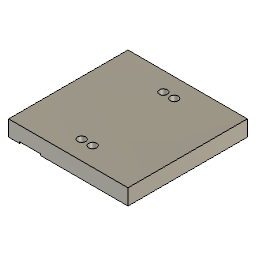
sample_stage (Autodesk Fusion 360 design; units mm, degrees)
part number: 2025-09-14-20-17-25-406
Autodesk Fusion 360 part; units mm, degrees
sketch "Sketch1" plane through (0, 0, 0) normal (0, 1, 0) x (1, 0, 0)
  line L0 (-30, -4) -> (30, -4)
  line L1 (30, -4) -> (30, 4)
  line L2 (30, 4) -> (-30, 4)
  line L3 (-30, 4) -> (-30, -4)
  line L4 (-30, -4) -> (30, 4) construction
  line L5 (30, -4) -> (-30, 4) construction
  line L6 (-30, 4) -> (-20, 4)
  line L7 (-20, 4) -> (-20, 14.75)
  line L8 (-20, 14.75) -> (-30, 14.75)
  line L9 (-30, 14.75) -> (-30, 4)
  line L10 (30, 4) -> (20, 4)
  line L11 (20, 4) -> (20, 14.75)
  line L12 (20, 14.75) -> (30, 14.75)
  line L13 (30, 14.75) -> (30, 4)
  dimension "d1" = 8
  dimension "d2" = 18.75
  dimension "d4" = 10
  dimension "d23" = 60
  constraint horizontal L0
  constraint perpendicular L0 L1
  constraint parallel L0 L2
  constraint parallel L1 L3
  constraint coincident L4 origin
  constraint coincident L5 origin
  constraint horizontal L6
  constraint vertical L7
  constraint horizontal L8
  constraint vertical L9
  constraint horizontal L10
  constraint vertical L11
  constraint horizontal L12
  constraint vertical L13
  constraint equal L8 L12
  constraint equal L9 L11
  measures "d1" distance of L0.end L1.end
  measures "d2" distance of L0 L12
  measures "d4" distance of L11.end L12.end
  measures "d23" distance of L0.start L0.end
extrude "Extrude1" add sketch "Sketch1" along normal mid plane 60 contours L0 L1 L2 L3 L6 L10
sketch "Sketch2" plane through (0, 0, 4) normal (0, 0, 1) x (-1, 0, 0)
  line L0 (-30, 30) -> (-30, -30)
  line L1 (-30, -30) -> (30, -30)
  line L2 (30, -30) -> (30, 30)
  line L3 (30, 30) -> (-30, 30)
  circle A0 centre (2.75, -20.5) radius 1.125
  circle A1 centre (-2.75, -20.5) radius 1.125
  circle A2 centre (2.75, 20.5) radius 1.125
  circle A3 centre (-2.75, 20.5) radius 1.125
  dimension "d8" = 2.25
  dimension "d9" = 41
  dimension "d10" = 20.5
  dimension "d11" = 5.5
  dimension "d12" = 2.75
  constraint horizontal A0.centre A1.centre
  constraint vertical A1.centre A3.centre
  constraint horizontal A2.centre A3.centre
  constraint vertical A0.centre A2.centre
  constraint equal A0 A1
  constraint equal A1 A3
  constraint equal A2 A3
  measures "d8" diameter of A3
  measures "d9" distance of A1.centre A3.centre
  measures "d10" vertical distance of origin A1.centre
  measures "d11" distance of A0.centre A1.centre
  measures "d12" horizontal distance of origin A1.centre
extrude "Extrude2" cut sketch "Sketch2" against normal up to surface (8 mm away) contours A0 | A1 | A2 | A3
sketch "Sketch3" plane through (0, -30, 0) normal (0, -1, 0) x (1, 0, 0)
  line L0 (-30, 4) -> (-30, -4)
  line L1 (-30, -4) -> (30, -4)
  line L2 (30, -4) -> (30, 4)
  line L3 (30, 4) -> (-30, 4)
  line L4 (-24.5, -4) -> (-14, -4)
  line L5 (-14, -4) -> (-14, -3.25)
  line L6 (-14, -3.25) -> (-24.5, -3.25)
  line L7 (-24.5, -3.25) -> (-24.5, -4)
  line L8 (30, -4) -> (22, -4)
  line L9 (22, -4) -> (22, -2.5)
  line L10 (22, -2.5) -> (30, -2.5)
  line L11 (30, -2.5) -> (30, -4)
  dimension "d24" = 10.5
  dimension "d27" = 0.75
  dimension "d28" = 5.5
  dimension "d33" = 8
  dimension "d34" = 1.5
  constraint horizontal L4
  constraint vertical L5
  constraint horizontal L6
  constraint vertical L7
  constraint coincident L1 L4.start
  constraint horizontal L8
  constraint vertical L9
  constraint horizontal L10
  constraint vertical L11
  constraint coincident L1.end L2.start
  measures "d24" distance of L5.end L6.end
  measures "d27" distance of L4.start L6.end
  measures "d28" distance of L0 L6.end
  measures "d33" distance of L9.end L10.end
  measures "d34" distance of L8.end L9.end
extrude "Extrude3" cut sketch "Sketch3" against normal blind 60 contours L1 L4 L5 L6 L7
sketch "Sketch4" plane through (0, 0, 4) normal (0, 0, 1) x (-1, 0, 0)
  circle A0 centre (-2.75, -20.5) radius 1.125
  circle A1 centre (-2.75, 20.5) radius 1.125
  circle A2 centre (2.75, -20.5) radius 1.125
  circle A3 centre (2.75, 20.5) radius 1.125
  line L0 (-30, 30) -> (-30, -30)
  line L1 (-30, -30) -> (30, -30)
  line L2 (30, -30) -> (30, 30)
  line L3 (30, 30) -> (-30, 30)
  circle A4 centre (-2.75, 20.5) radius 1.125
  circle A5 centre (2.75, 20.5) radius 1.125
  circle A6 centre (2.75, -20.5) radius 1.125
  circle A7 centre (-2.75, -20.5) radius 1.125
  circle A8 centre (-2.75, 20.5) radius 2
  circle A9 centre (2.75, 20.5) radius 2
  circle A10 centre (2.75, -20.5) radius 2
  circle A11 centre (-2.75, -20.5) radius 2
  dimension "d35" = 4
  constraint concentric A1 A8
  constraint concentric A3 A9
  constraint concentric A2 A10
  constraint concentric A7 A11
  constraint equal A10 A11
  constraint equal A9 A10
  constraint equal A8 A9
  measures "d35" diameter of A8
extrude "Extrude4" cut sketch "Sketch4" against normal blind 4.5 contours A8 | A9 | A10 | A11
sketch "Sketch5" plane through (0, -27.0005, 0) normal (0, 1, 0) x (-1, 0, 0)
  line L0 (-13.5, -11.5) -> (-10, -11.5)
  line L1 (-10.4635, -9.7651) -> (-12.4256, -9.7651)
  line L2 (-12.4256, -9.7651) -> (-12.4256, -11.6638)
  line L3 (-12.4256, -11.6638) -> (-10.4635, -11.6638)
  line L4 (-10.4635, -11.6638) -> (-10.4635, -9.7651)
  constraint horizontal L1
  constraint vertical L2
  constraint horizontal L3
  constraint vertical L4
sketch "Sketch7" plane through (0, 0, -17.4125) normal (0, 0, 1) x (-1, 0, 0)
  circle A0 centre (16.1, 33.84) radius 0.5
  circle A1 centre (8.48, 33.84) radius 0.5
  circle A2 centre (16.1, 31.3) radius 0.5
  circle A3 centre (8.48, 31.3) radius 0.5
  circle A4 centre (18.64, 31.3) radius 0.5
  circle A5 centre (11.02, 33.84) radius 0.5
  circle A6 centre (21.18, 33.84) radius 0.5
  circle A7 centre (18.64, 33.84) radius 0.5
  circle A8 centre (23.72, 31.3) radius 0.5
  circle A9 centre (13.56, 31.3) radius 0.5
  circle A10 centre (11.02, 31.3) radius 0.5
  circle A11 centre (21.18, 31.3) radius 0.5
  circle A12 centre (13.56, 33.84) radius 0.5
  circle A13 centre (23.72, 33.84) radius 0.5
  circle A14 centre (26.7, 45) radius 1.5875
  circle A15 centre (5.5, 45) radius 1.5875
  line L0 (29.75, 55.5) -> (2.45, 55.5)
  line L1 (2.45, 55.5) -> (2.45, 29.3)
  line L2 (2.45, 29.3) -> (29.75, 29.3)
  line L3 (29.75, 29.3) -> (29.75, 55.5)
  line L4 (7.5632, 31.2786) -> (4.5, 31.2786)
  line L5 (4.5, 31.2786) -> (4.5, 34)
  line L6 (4.5, 34) -> (7.5632, 34)
  line L7 (7.5632, 34) -> (7.5632, 31.2786)
  constraint horizontal L4
  constraint vertical L5
  constraint horizontal L6
  constraint vertical L7
sketch "Sketch8" plane through (0, 0, -17.4) normal (0, 0, 1) x (-1, 0, 0)
  line L0 (0, 17) -> (0, 45)
  line L1 (0, 45) -> (-22, 45)
  line L2 (-22, 45) -> (-22, 17)
  line L3 (-22, 17) -> (0, 17)
  line L4 (-8.4, 26.65) -> (-8.4, 22.35)
  line L5 (-8.4, 22.35) -> (-13.6, 22.35)
  line L6 (-13.6, 22.35) -> (-13.6, 26.65)
  line L7 (-13.6, 26.65) -> (-8.4, 26.65)
  circle A0 centre (-19.89, 39.26) radius 0.5
  circle A1 centre (-2.11, 39.26) radius 0.5
  circle A2 centre (-4.65, 39.26) radius 0.5
  circle A3 centre (-7.19, 39.26) radius 0.5
  circle A4 centre (-9.73, 39.26) radius 0.5
  circle A5 centre (-12.27, 39.26) radius 0.5
  circle A6 centre (-14.81, 39.26) radius 0.5
  circle A7 centre (-17.35, 39.26) radius 0.5
  circle A8 centre (-2.11, 41.8) radius 0.5
  circle A9 centre (-4.65, 41.8) radius 0.5
  circle A10 centre (-7.19, 41.8) radius 0.5
  circle A11 centre (-9.73, 41.8) radius 0.5
  circle A12 centre (-12.27, 41.8) radius 0.5
  circle A13 centre (-14.81, 41.8) radius 0.5
  circle A14 centre (-17.35, 41.8) radius 0.5
  circle A15 centre (-19.89, 41.8) radius 0.5
  circle A16 centre (-2, 30) radius 1.3
  circle A17 centre (-2, 19) radius 1.3
  circle A18 centre (-20, 19) radius 1.3
  circle A19 centre (-20, 30) radius 1.3
  line L8 (7.2208, 52.4505) -> (3.3661, 52.4505)
  line L9 (3.3661, 52.4505) -> (3.3661, 56.6136)
  line L10 (3.3661, 56.6136) -> (7.2208, 56.6136)
  line L11 (7.2208, 56.6136) -> (7.2208, 52.4505)
  line L12 (-0.0261, 52.4505) -> (-3.8808, 52.4505)
  line L13 (-3.8808, 52.4505) -> (-3.8808, 56.4594)
  line L14 (-3.8808, 56.4594) -> (-0.0261, 56.4594)
  line L15 (-0.0261, 56.4594) -> (-0.0261, 52.4505)
  constraint horizontal L8
  constraint vertical L9
  constraint horizontal L10
  constraint vertical L11
  constraint horizontal L12
  constraint vertical L13
  constraint horizontal L14
  constraint vertical L15
sketch "Sketch6" plane through (0, -16.6367, 0) normal (0, -1, 0) x (1, 0, 0)
  circle A0 centre (12.9741, -8.325) radius 0.35
  circle A1 through (-8.98, -17.4125, 14.6633) (-8.23, -17.4125, 15.0963) (-8.23, -17.4125, 14.2303)
  spline S0 degree 5 poles (12.9741, -8.325, 0) (12.9506, -8.4666, 0.3393) (12.9051, -8.7474, 1.064) (12.8415, -9.1609, 2.2899) (12.7658, -9.6969, 4.2025) (12.6803, -10.3411, 7.0535) (12.5848, -10.9583, 10.3471) (12.4405, -11.5467, 14.0424) (12.1824, -12.1037, 18.0652) (11.7132, -12.6253, 22.2988) (10.9253, -13.1066, 26.5936) (9.7213, -13.5411, 30.7741) (8.0349, -13.921, 34.6474) (5.8533, -14.2365, 38.0098) (3.2361, -14.4766, 40.6561) (0.3449, -14.6277, 42.3847) (-2.5543, -14.6756, 43.0126) (-5.1645, -14.6125, 42.4121) (-7.2194, -14.4435, 40.5466) (-8.5459, -14.193, 37.5053) (-9.1365, -13.913, 33.5472) (-9.1137, -13.6749, 29.0548) (-8.6842, -13.5604, 24.4779) (-8.0984, -13.6527, 20.2834) (-7.6062, -14.0278, 16.9005) (-7.4198, -14.7459, 14.6739) (-7.6129, -15.6209, 13.9709) (-7.9657, -16.4497, 14.0728) (-8.2932, -17.0788, 14.42) (-8.48, -17.4125, 14.6633) knots 0 0 0 0 0 0 0.04 0.08 0.12 0.16 0.2 0.24 0.28 0.32 0.36 0.4 0.44 0.48 0.52 0.56 0.6 0.64 0.68 0.72 0.76 0.8 0.84 0.88 0.92 0.96 1 1 1 1 1 1
  line L0 (-7.5632, -14.4125, 14.6419) -> (-7.5632, -14.4125, 17.3633)
  point P0 (-7.5632, -14.4125)
  point P1 (3.8808, -14.4)
  point P2 (-7.2208, -14.4)
  point P3 (12.4256, -11.5)
  point P4 (12.4256, -11.5)
  point P5 (3.8808, -14.4)
  point P6 (-7.2208, -14.4)
  point P7 (-7.5632, -14.4125)
  constraint coincident P4 P3
  constraint coincident P5 P1
  constraint coincident P6 P2
sketch "Sketch9" plane through (0, 0, -5.15) normal (0, 0, 1) x (-1, 0, 0)
  circle A0 centre (-24.5, 10.2805) radius 1.25
  circle A1 centre (-24.5, 25.2805) radius 1.25
  line L0 (-21, 11.7505) -> (-21, 24.5005)
  arc A2 (-22, 25.5005) -> (-21, 24.5005) centre (-21, 25.5005) ccw
  line L1 (-22, 25.5005) -> (-22, 27.0005)
  arc A3 (-20, 27.0005) -> (-22, 27.0005) centre (-21, 27.0005) ccw
  line L2 (-20, 27.0005) -> (-18.5, 27.0005)
  arc A4 (-18.5, 23.0005) -> (-18.5, 27.0005) centre (-18.5, 25.0005) ccw
  line L3 (-18.5, 23.0005) -> (-18.9866, 23.0005)
  line L4 (-18.9866, 23.0005) -> (-18.9866, 21.5005)
  line L5 (-18.9866, 21.5005) -> (-13.0134, 21.5005)
  line L6 (-13.0134, 21.5005) -> (-13.0134, 23.0005)
  line L7 (-13.0134, 23.0005) -> (-13.5, 23.0005)
  arc A5 (-13.5, 27.0005) -> (-13.5, 23.0005) centre (-13.5, 25.0005) ccw
  line L8 (-13.5, 27.0005) -> (-10, 27.0005)
  line L9 (-10, 27.0005) -> (-10, 9.5605)
  line L10 (-10, 9.5605) -> (-8, 9.5605)
  arc A6 (-8, 9.5605) -> (-8, 11.5605) centre (-8, 10.5605) ccw
  line L11 (-8, 11.5605) -> (-8, 30.0005)
  line L12 (-8, 30.0005) -> (-20, 30.0005)
  arc A7 (-22, 30.0005) -> (-20, 30.0005) centre (-21, 30.0005) ccw
  line L13 (-22, 30.0005) -> (-27, 30.0005)
  line L14 (-27, 30.0005) -> (-27, 5.5605)
  line L15 (-27, 5.5605) -> (-13.0134, 5.5605)
  line L16 (-13.0134, 5.5605) -> (-13.0134, 11.7505)
  line L17 (-13.0134, 11.7505) -> (-21, 11.7505)
  line L18 (-18.1647, 30.0005) -> (-19.25, 30.0005)
  line L19 (-19.25, 30.0005) -> (-19.25, 25.4822)
  line L20 (-19.25, 25.4822) -> (-18.1647, 25.4822)
  line L21 (-18.1647, 25.4822) -> (-18.1647, 30.0005)
  constraint horizontal L18
  constraint vertical L19
  constraint horizontal L20
  constraint vertical L21
  constraint coincident L12 L18.start
sketch "Sketch10" plane through (0, -16.6367, 0) normal (0, -1, 0) x (1, 0, 0)
  circle A0 centre (19.0259, -8.325) radius 0.35
  circle A1 through (-8.98, -17.4125, 17.2033) (-8.23, -17.4125, 17.6363) (-8.23, -17.4125, 16.7703)
  spline S0 degree 5 poles (19.0259, -8.325, 0) (19.2072, -8.4658, 0.3949) (19.5347, -8.7445, 1.212) (19.9208, -9.1539, 2.5199) (20.2248, -9.6823, 4.4288) (20.2496, -10.3134, 7.0879) (19.9136, -10.9144, 10.0105) (19.2098, -11.4843, 13.1738) (18.1304, -12.0219, 16.5367) (16.6677, -12.5256, 20.0336) (14.8204, -12.993, 23.5767) (12.6004, -13.4205, 27.0581) (10.0402, -13.8027, 30.3511) (7.1997, -14.1321, 33.3127) (4.1743, -14.3984, 35.7844) (1.1023, -14.5883, 37.595) (-1.8247, -14.6845, 38.5598) (-4.3972, -14.6728, 38.5184) (-6.4305, -14.5499, 37.3777) (-7.8004, -14.3306, 35.1495) (-8.4925, -14.0577, 32.0033) (-8.616, -13.8034, 28.2757) (-8.3545, -13.6552, 24.3947) (-7.9324, -13.7064, 20.826) (-7.5739, -14.0434, 18.0081) (-7.4695, -14.736, 16.2994) (-7.6766, -15.6052, 15.9801) (-8.0094, -16.4384, 16.3536) (-8.31, -17.0744, 16.8747) (-8.48, -17.4125, 17.2033) knots 0 0 0 0 0 0 0.04 0.08 0.12 0.16 0.2 0.24 0.28 0.32 0.36 0.4 0.44 0.48 0.52 0.56 0.6 0.64 0.68 0.72 0.76 0.8 0.84 0.88 0.92 0.96 1 1 1 1 1 1
  line L0 (20, -11.5, 13.3638) -> (8, -11.5, 13.3638)
  point P0 (18.1647, -4.65)
  point P1 (18.1647, -4.65)
  point P2 (3.8808, -14.4)
  point P3 (-7.2208, -14.4)
  point P4 (-7.5632, -14.4125)
  point P5 (20, -11.5)
  point P6 (19.0772, -11.5)
  point P7 (3.8808, -14.4)
  point P8 (-7.2208, -14.4)
  point P9 (-7.5632, -14.4125)
  constraint coincident P7 P2
  constraint coincident P8 P3
  constraint coincident P9 P4
sketch "Sketch11" plane through (0, 0, -15.4) normal (0, 0, 1) x (-1, 0, 0)
  circle A0 centre (-2.11, 39.26) radius 0.35
  circle A1 centre (-7.19, 39.26) radius 0.35
  line L0 (-7.19, 39.26, 0) -> (-7.19, 39.26, 0.2831)
  line L1 (-7.19, 39.76, 0.7831) -> (-7.19, 42.9444, 0.7831)
  line L2 (-7.19, 42.9444, 0.7831) -> (-7.19, 47.4223, 0.7831)
  line L3 (-7.19, 47.4223, 0.7831) -> (-7.19, 49.3647, 0.7831)
  line L4 (-6.69, 49.8647, 0.7831) -> (9.3272, 49.8647, 0.7831)
  line L5 (9.3272, 49.8647, 0.7831) -> (18.14, 49.8647, 0.7831)
  line L6 (29.75, 55.5, -2.0125) -> (29.75, 55.5, -3.6)
  arc A2 through (-7.19, 39.26, 0.2831) (-7.19, 39.4064, 0.6367) (-7.19, 39.76, 0.7831)
  arc A3 through (-6.69, 49.8647, 0.7831) (-7.0436, 49.7182, 0.7831) (-7.19, 49.3647, 0.7831)
  line L7 (18.64, 49.3647, 0.7831) -> (18.64, 34.34, 0.7831)
  line L8 (18.64, 33.84, 0.2831) -> (18.64, 33.84, -0.6)
  line L9 (29.75, 29.3, -2.0125) -> (29.75, 29.3, -3.6)
  arc A4 through (18.64, 33.84, 0.2831) (18.64, 33.9864, 0.6367) (18.64, 34.34, 0.7831)
  arc A5 through (18.64, 49.3647, 0.7831) (18.4936, 49.7182, 0.7831) (18.14, 49.8647, 0.7831)
  circle A6 through (21.53, 31.3, -0.6) (21.005, 31.6031, -0.6) (21.005, 30.9969, -0.6)
  circle A7 through (16.45, 31.3, -0.6) (15.925, 31.6031, -0.6) (15.925, 30.9969, -0.6)
  circle A8 through (11.37, 33.84, -0.6) (10.845, 34.1431, -0.6) (10.845, 33.5369, -0.6)
  circle A9 through (13.91, 31.3, -0.6) (13.385, 31.6031, -0.6) (13.385, 30.9969, -0.6)
  circle A10 through (21.53, 33.84, -0.6) (21.005, 34.1431, -0.6) (21.005, 33.5369, -0.6)
  circle A11 through (13.91, 33.84, -0.6) (13.385, 34.1431, -0.6) (13.385, 33.5369, -0.6)
  circle A12 through (8.83, 33.84, -0.6) (8.305, 34.1431, -0.6) (8.305, 33.5369, -0.6)
  circle A13 through (18.99, 33.84, -0.6) (18.465, 34.1431, -0.6) (18.465, 33.5369, -0.6)
  circle A14 through (8.83, 31.3, -0.6) (8.305, 31.6031, -0.6) (8.305, 30.9969, -0.6)
  circle A15 through (11.37, 31.3, -0.6) (10.845, 31.6031, -0.6) (10.845, 30.9969, -0.6)
  circle A16 through (24.07, 33.84, -0.6) (23.545, 34.1431, -0.6) (23.545, 33.5369, -0.6)
  circle A17 through (16.45, 33.84, -0.6) (15.925, 34.1431, -0.6) (15.925, 33.5369, -0.6)
  circle A18 through (18.99, 31.3, -0.6) (18.465, 31.6031, -0.6) (18.465, 30.9969, -0.6)
  circle A19 through (24.07, 31.3, -0.6) (23.545, 31.6031, -0.6) (23.545, 30.9969, -0.6)
  point P0 (-6.84, 39.26)
  point P1 (11.37, 33.84)
  point P2 (8.83, 31.3)
  point P3 (21.53, 31.3)
  point P4 (24.07, 31.3)
  point P5 (8.83, 33.84)
  point P6 (13.91, 31.3)
  point P7 (21.53, 33.84)
  point P8 (24.07, 33.84)
  point P9 (16.45, 31.3)
  point P10 (13.91, 33.84)
  point P11 (11.37, 31.3)
  point P12 (16.45, 33.84)
  point P13 (18.99, 33.84)
  point P14 (18.99, 31.3)
  dimension "d67" = 0.5
  dimension "d68" = 0.5
  dimension "d70" = 0.5
  dimension "d71" = 0.5
sketch "Sketch12" plane through (0, 0, -15.4) normal (0, 0, 1) x (-1, 0, 0)
  circle A0 centre (-4.65, 39.26) radius 0.35
  line L0 (-4.65, 39.26, 0) -> (-4.65, 39.26, 0.2958)
  line L1 (-4.65, 39.76, 0.7958) -> (-4.65, 46.3677, 0.7958)
  line L2 (-3.65, 47.3677, 0.7958) -> (2.35, 47.3677, 0.7958)
  line L3 (2.35, 47.3677, 0.7958) -> (15.1, 47.3677, 0.7958)
  line L4 (16.1, 46.3677, 0.7958) -> (16.1, 34.34, 0.7958)
  line L5 (16.1, 33.84, 0.2958) -> (16.1, 33.84, -0.6)
  line L6 (29.75, 29.3, -2.0125) -> (29.75, 29.3, -3.6)
  arc A1 through (16.1, 46.3677, 0.7958) (15.8071, 47.0749, 0.7958) (15.1, 47.3677, 0.7958)
  arc A2 through (-3.65, 47.3677, 0.7958) (-4.3571, 47.0749, 0.7958) (-4.65, 46.3677, 0.7958)
  arc A3 through (-4.65, 39.76, 0.7958) (-4.65, 39.4064, 0.6493) (-4.65, 39.26, 0.2958)
  arc A4 through (16.1, 33.84, 0.2958) (16.1, 33.9864, 0.6493) (16.1, 34.34, 0.7958)
  circle A5 through (21.53, 31.3, -0.6) (21.005, 31.6031, -0.6) (21.005, 30.9969, -0.6)
  circle A6 through (16.45, 31.3, -0.6) (15.925, 31.6031, -0.6) (15.925, 30.9969, -0.6)
  circle A7 through (11.37, 33.84, -0.6) (10.845, 34.1431, -0.6) (10.845, 33.5369, -0.6)
  circle A8 through (13.91, 31.3, -0.6) (13.385, 31.6031, -0.6) (13.385, 30.9969, -0.6)
  circle A9 through (21.53, 33.84, -0.6) (21.005, 34.1431, -0.6) (21.005, 33.5369, -0.6)
  circle A10 through (13.91, 33.84, -0.6) (13.385, 34.1431, -0.6) (13.385, 33.5369, -0.6)
  circle A11 through (8.83, 33.84, -0.6) (8.305, 34.1431, -0.6) (8.305, 33.5369, -0.6)
  circle A12 through (18.99, 33.84, -0.6) (18.465, 34.1431, -0.6) (18.465, 33.5369, -0.6)
  circle A13 through (8.83, 31.3, -0.6) (8.305, 31.6031, -0.6) (8.305, 30.9969, -0.6)
  circle A14 through (11.37, 31.3, -0.6) (10.845, 31.6031, -0.6) (10.845, 30.9969, -0.6)
  circle A15 through (24.07, 33.84, -0.6) (23.545, 34.1431, -0.6) (23.545, 33.5369, -0.6)
  circle A16 through (16.45, 33.84, -0.6) (15.925, 34.1431, -0.6) (15.925, 33.5369, -0.6)
  circle A17 through (18.99, 31.3, -0.6) (18.465, 31.6031, -0.6) (18.465, 30.9969, -0.6)
  circle A18 through (24.07, 31.3, -0.6) (23.545, 31.6031, -0.6) (23.545, 30.9969, -0.6)
  dimension "d72" = 1
  dimension "d79" = 1
sketch "Sketch13" plane through (0, 0, -15.4) normal (0, 0, 1) x (-1, 0, 0)
  circle A0 centre (-2.11, 39.26) radius 0.35
  line L0 (-2.11, 39.26, 0) -> (-2.11, 39.26, 0.2304)
  line L1 (-2.11, 39.76, 0.7304) -> (-2.11, 44.4826, 0.7304)
  line L2 (-1.61, 44.9826, 0.7304) -> (13.06, 44.9826, 0.7304)
  line L3 (13.56, 44.4826, 0.7304) -> (13.56, 34.34, 0.7304)
  line L4 (13.56, 33.84, 0.2304) -> (13.56, 33.84, -0.6)
  line L5 (29.75, 29.3, -2.0125) -> (29.75, 29.3, -3.6)
  arc A1 through (13.56, 33.84, 0.2304) (13.56, 33.9864, 0.5839) (13.56, 34.34, 0.7304)
  arc A2 through (13.56, 44.4826, 0.7304) (13.4136, 44.8361, 0.7304) (13.06, 44.9826, 0.7304)
  arc A3 through (-1.61, 44.9826, 0.7304) (-1.9636, 44.8361, 0.7304) (-2.11, 44.4826, 0.7304)
  arc A4 through (-2.11, 39.26, 0.2304) (-2.11, 39.4064, 0.5839) (-2.11, 39.76, 0.7304)
  circle A5 through (21.53, 31.3, -0.6) (21.005, 31.6031, -0.6) (21.005, 30.9969, -0.6)
  circle A6 through (16.45, 31.3, -0.6) (15.925, 31.6031, -0.6) (15.925, 30.9969, -0.6)
  circle A7 through (11.37, 33.84, -0.6) (10.845, 34.1431, -0.6) (10.845, 33.5369, -0.6)
  circle A8 through (13.91, 31.3, -0.6) (13.385, 31.6031, -0.6) (13.385, 30.9969, -0.6)
  circle A9 through (21.53, 33.84, -0.6) (21.005, 34.1431, -0.6) (21.005, 33.5369, -0.6)
  circle A10 through (13.91, 33.84, -0.6) (13.385, 34.1431, -0.6) (13.385, 33.5369, -0.6)
  circle A11 through (8.83, 33.84, -0.6) (8.305, 34.1431, -0.6) (8.305, 33.5369, -0.6)
  circle A12 through (18.99, 33.84, -0.6) (18.465, 34.1431, -0.6) (18.465, 33.5369, -0.6)
  circle A13 through (8.83, 31.3, -0.6) (8.305, 31.6031, -0.6) (8.305, 30.9969, -0.6)
  circle A14 through (11.37, 31.3, -0.6) (10.845, 31.6031, -0.6) (10.845, 30.9969, -0.6)
  circle A15 through (24.07, 33.84, -0.6) (23.545, 34.1431, -0.6) (23.545, 33.5369, -0.6)
  circle A16 through (16.45, 33.84, -0.6) (15.925, 34.1431, -0.6) (15.925, 33.5369, -0.6)
  circle A17 through (18.99, 31.3, -0.6) (18.465, 31.6031, -0.6) (18.465, 30.9969, -0.6)
  circle A18 through (24.07, 31.3, -0.6) (23.545, 31.6031, -0.6) (23.545, 30.9969, -0.6)
  dimension "d80" = 0.5
sketch "Sketch14" plane through (0, 0, -3.9) normal (0, 0, 1) x (-1, 0, 0)
  line L0 (33.2443, 31.3, -4.9763) -> (14.0837, 31.3, -4.9763)
  line L1 (13.56, 31.3, -5.5) -> (13.56, 31.3, -12.1)
  line L2 (7.6, 30, -8.1) -> (7.6, 30, -3.6)
  arc A0 through (13.56, 31.3, -5.5) (13.7134, 31.3, -5.1297) (14.0837, 31.3, -4.9763)
  line L3 (33.7443, 30.8, -4.9763) -> (33.7443, 1.8, -4.9763)
  line L4 (33.7443, 1.3, -4.4763) -> (33.7443, 1.3, -2.4216)
  arc A1 through (33.7443, 30.8, -4.9763) (33.5979, 31.1536, -4.9763) (33.2443, 31.3, -4.9763)
  arc A2 through (33.7443, 1.3, -4.4763) (33.7443, 1.4464, -4.8298) (33.7443, 1.8, -4.9763)
  circle A3 through (21.53, 31.3, -12.1) (21.005, 31.6031, -12.1) (21.005, 30.9969, -12.1)
  circle A4 through (16.45, 31.3, -12.1) (15.925, 31.6031, -12.1) (15.925, 30.9969, -12.1)
  circle A5 through (11.37, 33.84, -12.1) (10.845, 34.1431, -12.1) (10.845, 33.5369, -12.1)
  circle A6 through (13.91, 31.3, -12.1) (13.385, 31.6031, -12.1) (13.385, 30.9969, -12.1)
  circle A7 through (21.53, 33.84, -12.1) (21.005, 34.1431, -12.1) (21.005, 33.5369, -12.1)
  circle A8 through (13.91, 33.84, -12.1) (13.385, 34.1431, -12.1) (13.385, 33.5369, -12.1)
  circle A9 through (8.83, 33.84, -12.1) (8.305, 34.1431, -12.1) (8.305, 33.5369, -12.1)
  circle A10 through (18.99, 33.84, -12.1) (18.465, 34.1431, -12.1) (18.465, 33.5369, -12.1)
  circle A11 through (8.83, 31.3, -12.1) (8.305, 31.6031, -12.1) (8.305, 30.9969, -12.1)
  circle A12 through (11.37, 31.3, -12.1) (10.845, 31.6031, -12.1) (10.845, 30.9969, -12.1)
  circle A13 through (24.07, 33.84, -12.1) (23.545, 34.1431, -12.1) (23.545, 33.5369, -12.1)
  circle A14 through (16.45, 33.84, -12.1) (15.925, 34.1431, -12.1) (15.925, 33.5369, -12.1)
  circle A15 through (18.99, 31.3, -12.1) (18.465, 31.6031, -12.1) (18.465, 30.9969, -12.1)
  circle A16 through (24.07, 31.3, -12.1) (23.545, 31.6031, -12.1) (23.545, 30.9969, -12.1)
  dimension "d108" = 0.5
sketch "Sketch15" plane through (0, 0, -3.9) normal (0, 0, 1) x (-1, 0, 0)
  line L0 (33.3467, 31.3, -6.5145) -> (16.6, 31.3, -6.5145)
  line L1 (16.1, 31.3, -7.0145) -> (16.1, 31.3, -12.1)
  arc A0 through (16.1, 31.3, -7.0145) (16.2464, 31.3, -6.661) (16.6, 31.3, -6.5145)
  line L2 (33.8467, 30.8, -6.5145) -> (33.8467, -0.6852, -6.5145)
  line L3 (33.8467, -1.1852, -6.0145) -> (33.8467, -1.1852, -2.8897)
  arc A1 through (33.8467, 30.8, -6.5145) (33.7003, 31.1536, -6.5145) (33.3467, 31.3, -6.5145)
  arc A2 through (33.8467, -0.6852, -6.5145) (33.8467, -1.0387, -6.3681) (33.8467, -1.1852, -6.0145)
  dimension "d94" = 0.5
  dimension "d109" = 0.5
sketch "Sketch16" plane through (0, 0, -3.9) normal (0, 0, 1) x (-1, 0, 0)
  line L0 (33.3217, 31.3, -8.1959) -> (19.3169, 31.3, -8.1959)
  line L1 (18.64, 31.3, -8.8729) -> (18.64, 31.3, -12.1)
  arc A0 through (19.3169, 31.3, -8.1959) (18.8383, 31.3, -8.3942) (18.64, 31.3, -8.8729)
  line L2 (33.8217, 30.8, -8.1959) -> (33.8217, -3.328, -8.1959)
  line L3 (33.8217, -3.828, -7.6959) -> (33.8217, -3.828, -2.6955)
  arc A1 through (33.8217, 30.8, -8.1959) (33.6753, 31.1536, -8.1959) (33.3217, 31.3, -8.1959)
  arc A2 through (33.8217, -3.828, -7.6959) (33.8217, -3.6815, -8.0495) (33.8217, -3.328, -8.1959)
  circle A3 through (21.53, 31.3, -12.1) (21.005, 31.6031, -12.1) (21.005, 30.9969, -12.1)
  circle A4 through (16.45, 31.3, -12.1) (15.925, 31.6031, -12.1) (15.925, 30.9969, -12.1)
  circle A5 through (11.37, 33.84, -12.1) (10.845, 34.1431, -12.1) (10.845, 33.5369, -12.1)
  circle A6 through (13.91, 31.3, -12.1) (13.385, 31.6031, -12.1) (13.385, 30.9969, -12.1)
  circle A7 through (21.53, 33.84, -12.1) (21.005, 34.1431, -12.1) (21.005, 33.5369, -12.1)
  circle A8 through (13.91, 33.84, -12.1) (13.385, 34.1431, -12.1) (13.385, 33.5369, -12.1)
  circle A9 through (8.83, 33.84, -12.1) (8.305, 34.1431, -12.1) (8.305, 33.5369, -12.1)
  circle A10 through (18.99, 33.84, -12.1) (18.465, 34.1431, -12.1) (18.465, 33.5369, -12.1)
  circle A11 through (8.83, 31.3, -12.1) (8.305, 31.6031, -12.1) (8.305, 30.9969, -12.1)
  circle A12 through (11.37, 31.3, -12.1) (10.845, 31.6031, -12.1) (10.845, 30.9969, -12.1)
  circle A13 through (24.07, 33.84, -12.1) (23.545, 34.1431, -12.1) (23.545, 33.5369, -12.1)
  circle A14 through (16.45, 33.84, -12.1) (15.925, 34.1431, -12.1) (15.925, 33.5369, -12.1)
  circle A15 through (18.99, 31.3, -12.1) (18.465, 31.6031, -12.1) (18.465, 30.9969, -12.1)
  circle A16 through (24.07, 31.3, -12.1) (23.545, 31.6031, -12.1) (23.545, 30.9969, -12.1)
  dimension "d110" = 0.5
sketch "Sketch17" plane through (0, 0, -16) normal (0, 0, 1) x (-1, 0, 0)
  line L0 (21.68, 31.3, 2.5683) -> (33.2222, 31.3, 2.5683)
  line L1 (33.7222, 30.8, 2.5683) -> (33.7222, -5.7983, 2.5683)
  line L2 (33.7222, -6.2983, 3.0683) -> (33.7222, -6.2983, 9.4009)
  line L3 (21.18, 31.3, 0) -> (21.18, 31.3, 2.0683)
  arc A0 through (33.7222, 30.8, 2.5683) (33.5758, 31.1536, 2.5683) (33.2222, 31.3, 2.5683)
  arc A1 through (33.7222, -6.2983, 3.0683) (33.7222, -6.1518, 2.7147) (33.7222, -5.7983, 2.5683)
  arc A2 through (21.18, 31.3, 2.0683) (21.3264, 31.3, 2.4218) (21.68, 31.3, 2.5683)
  circle A3 centre (21.18, 31.3) radius 0.35
  circle A4 centre (16.1, 31.3) radius 0.35
  circle A5 centre (11.02, 33.84) radius 0.35
  circle A6 centre (13.56, 31.3) radius 0.35
  circle A7 centre (21.18, 33.84) radius 0.35
  circle A8 centre (13.56, 33.84) radius 0.35
  circle A9 centre (8.48, 33.84) radius 0.35
  circle A10 centre (18.64, 33.84) radius 0.35
  circle A11 centre (8.48, 31.3) radius 0.35
  circle A12 centre (11.02, 31.3) radius 0.35
  circle A13 centre (23.72, 33.84) radius 0.35
  circle A14 centre (16.1, 33.84) radius 0.35
  circle A15 centre (18.64, 31.3) radius 0.35
  circle A16 centre (23.72, 31.3) radius 0.35
  dimension "d117" = 0.5
  dimension "d124" = 0.5
sketch "Sketch18" plane through (0, 0, -16) normal (0, 0, 1) x (-1, 0, 0)
  line L0 (23.72, 31.3, 0) -> (23.72, 31.3, 0.7434)
  line L1 (24.22, 31.3, 1.2434) -> (33.2385, 31.3, 1.2434)
  line L2 (33.7385, 30.8, 1.2434) -> (33.7385, -8.4721, 1.2434)
  line L3 (33.7385, -8.9721, 1.7434) -> (33.7385, -8.9721, 9.6414)
  arc A0 through (24.22, 31.3, 1.2434) (23.8664, 31.3, 1.0969) (23.72, 31.3, 0.7434)
  arc A1 through (33.7385, 30.8, 1.2434) (33.5921, 31.1536, 1.2434) (33.2385, 31.3, 1.2434)
  arc A2 through (33.7385, -8.9721, 1.7434) (33.7385, -8.8256, 1.3898) (33.7385, -8.4721, 1.2434)
  circle A3 centre (21.18, 31.3) radius 0.35
  circle A4 centre (16.1, 31.3) radius 0.35
  circle A5 centre (11.02, 33.84) radius 0.35
  circle A6 centre (13.56, 31.3) radius 0.35
  circle A7 centre (21.18, 33.84) radius 0.35
  circle A8 centre (13.56, 33.84) radius 0.35
  circle A9 centre (8.48, 33.84) radius 0.35
  circle A10 centre (18.64, 33.84) radius 0.35
  circle A11 centre (8.48, 31.3) radius 0.35
  circle A12 centre (11.02, 31.3) radius 0.35
  circle A13 centre (23.72, 33.84) radius 0.35
  circle A14 centre (16.1, 33.84) radius 0.35
  circle A15 centre (18.64, 31.3) radius 0.35
  circle A16 centre (23.72, 31.3) radius 0.35
  dimension "d125" = 0.5
sketch "Sketch19" plane through (0, -16.6367, 0) normal (0, -1, 0) x (1, 0, 0)
  circle A0 centre (12.9741, -8.325) radius 0.35
  line L0 (12.9741, -8.325, 0) -> (12.9686, -8.325, 1.7366)
  line L1 (12.9654, -9.325, 2.7366) -> (12.9654, -10.75, 2.7366)
  line L2 (12.9654, -11.75, 3.7366) -> (12.9654, -11.75, 13.6633)
  line L3 (11.9654, -11.75, 14.6633) -> (-7.48, -11.75, 14.6633)
  line L4 (-8.48, -12.75, 14.6633) -> (-8.48, -16, 14.6633)
  arc A1 through (12.9654, -9.325, 2.7366) (12.9663, -8.6179, 2.4437) (12.9686, -8.325, 1.7366)
  arc A2 through (12.9654, -11.75, 3.7366) (12.9654, -11.4571, 3.0295) (12.9654, -10.75, 2.7366)
  arc A3 through (11.9654, -11.75, 14.6633) (12.6725, -11.75, 14.3704) (12.9654, -11.75, 13.6633)
  arc A4 through (-7.48, -11.75, 14.6633) (-8.1871, -12.0429, 14.6633) (-8.48, -12.75, 14.6633)
  circle A5 through (-20.83, -16, 14.6633) (-21.355, -16, 14.9664) (-21.355, -16, 14.3602)
  circle A6 through (-15.75, -16, 14.6633) (-16.275, -16, 14.9664) (-16.275, -16, 14.3602)
  circle A7 through (-10.67, -16, 17.2033) (-11.195, -16, 17.5064) (-11.195, -16, 16.9002)
  circle A8 through (-13.21, -16, 14.6633) (-13.735, -16, 14.9664) (-13.735, -16, 14.3602)
  circle A9 through (-20.83, -16, 17.2033) (-21.355, -16, 17.5064) (-21.355, -16, 16.9002)
  circle A10 through (-13.21, -16, 17.2033) (-13.735, -16, 17.5064) (-13.735, -16, 16.9002)
  circle A11 through (-8.13, -16, 17.2033) (-8.655, -16, 17.5064) (-8.655, -16, 16.9002)
  circle A12 through (-18.29, -16, 17.2033) (-18.815, -16, 17.5064) (-18.815, -16, 16.9002)
  circle A13 through (-8.13, -16, 14.6633) (-8.655, -16, 14.9664) (-8.655, -16, 14.3602)
  circle A14 through (-10.67, -16, 14.6633) (-11.195, -16, 14.9664) (-11.195, -16, 14.3602)
  circle A15 through (-23.37, -16, 17.2033) (-23.895, -16, 17.5064) (-23.895, -16, 16.9002)
  circle A16 through (-15.75, -16, 17.2033) (-16.275, -16, 17.5064) (-16.275, -16, 16.9002)
  circle A17 through (-18.29, -16, 14.6633) (-18.815, -16, 14.9664) (-18.815, -16, 14.3602)
  circle A18 through (-23.37, -16, 14.6633) (-23.895, -16, 14.9664) (-23.895, -16, 14.3602)
  dimension "d132" = 0.25
  dimension "d133" = 1
sketch "Sketch20" plane through (0, -16.6367, 0) normal (0, -1, 0) x (1, 0, 0)
  circle A0 centre (19.0259, -8.325) radius 0.35
  line L0 (19.0259, -8.325, 0) -> (19.0259, -8.325, 3.5)
  line L1 (19.0259, -8.825, 4) -> (19.0259, -11.25, 4)
  line L2 (19.0259, -11.75, 4.5) -> (19.0259, -11.75, 16.7033)
  line L3 (19.0259, -12.25, 17.2033) -> (19.0259, -12.325, 17.2033)
  line L4 (18.5259, -12.825, 17.2033) -> (-7.48, -12.825, 17.2033)
  line L5 (-8.48, -13.825, 17.2033) -> (-8.48, -16, 17.2033)
  arc A1 through (-7.48, -12.825, 17.2033) (-8.1871, -13.1179, 17.2033) (-8.48, -13.825, 17.2033)
  arc A2 through (18.5259, -12.825, 17.2033) (18.8795, -12.6786, 17.2033) (19.0259, -12.325, 17.2033)
  arc A3 through (19.0259, -12.25, 17.2033) (19.0259, -11.8964, 17.0569) (19.0259, -11.75, 16.7033)
  arc A4 through (19.0259, -11.75, 4.5) (19.0259, -11.6036, 4.1464) (19.0259, -11.25, 4)
  arc A5 through (19.0259, -8.825, 4) (19.0259, -8.4714, 3.8536) (19.0259, -8.325, 3.5)
  circle A6 through (-20.83, -16, 14.6633) (-21.355, -16, 14.9664) (-21.355, -16, 14.3602)
  circle A7 through (-15.75, -16, 14.6633) (-16.275, -16, 14.9664) (-16.275, -16, 14.3602)
  circle A8 through (-10.67, -16, 17.2033) (-11.195, -16, 17.5064) (-11.195, -16, 16.9002)
  circle A9 through (-13.21, -16, 14.6633) (-13.735, -16, 14.9664) (-13.735, -16, 14.3602)
  circle A10 through (-20.83, -16, 17.2033) (-21.355, -16, 17.5064) (-21.355, -16, 16.9002)
  circle A11 through (-13.21, -16, 17.2033) (-13.735, -16, 17.5064) (-13.735, -16, 16.9002)
  circle A12 through (-8.13, -16, 17.2033) (-8.655, -16, 17.5064) (-8.655, -16, 16.9002)
  circle A13 through (-18.29, -16, 17.2033) (-18.815, -16, 17.5064) (-18.815, -16, 16.9002)
  circle A14 through (-8.13, -16, 14.6633) (-8.655, -16, 14.9664) (-8.655, -16, 14.3602)
  circle A15 through (-10.67, -16, 14.6633) (-11.195, -16, 14.9664) (-11.195, -16, 14.3602)
  circle A16 through (-23.37, -16, 17.2033) (-23.895, -16, 17.5064) (-23.895, -16, 16.9002)
  circle A17 through (-15.75, -16, 17.2033) (-16.275, -16, 17.5064) (-16.275, -16, 16.9002)
  circle A18 through (-18.29, -16, 14.6633) (-18.815, -16, 14.9664) (-18.815, -16, 14.3602)
  circle A19 through (-23.37, -16, 14.6633) (-23.895, -16, 14.9664) (-23.895, -16, 14.3602)
  dimension "d140" = 0.25
  dimension "d141" = 1
  dimension "d142" = 0.5
sketch "Sketch21" plane through (-14.3562, 0, 0) normal (-1, 0, 0) x (0, -1, 0)
  circle A0 centre (-12.9741, -19.825) radius 0.35
  line L0 (-12.9741, -19.825, 0) -> (-12.9741, -19.825, 3.2188)
  line L1 (-12.9741, -20.325, 3.7188) -> (-12.9741, -22.25, 3.7188)
  line L2 (-12.9741, -22.75, 4.2188) -> (-12.9741, -22.75, 20.9824)
  line L3 (-12.9741, -22.25, 21.4824) -> (-12.9741, -12.5756, 21.4824)
  line L4 (-12.4741, -12.0756, 21.4824) -> (32.2346, -12.0756, 21.4824)
  line L5 (32.7346, -12.0756, 20.9824) -> (32.7346, -12.0756, -2.8362)
  line L6 (32.2346, -12.0756, -3.3362) -> (31.8, -12.0756, -3.3362)
  line L7 (31.3, -12.5756, -3.3362) -> (31.3, -16, -3.3362)
  arc A1 through (-12.9741, -22.75, 4.2188) (-12.9741, -22.6036, 3.8653) (-12.9741, -22.25, 3.7188)
  arc A2 through (-12.9741, -22.25, 21.4824) (-12.9741, -22.6036, 21.336) (-12.9741, -22.75, 20.9824)
  arc A3 through (-12.4741, -12.0756, 21.4824) (-12.8276, -12.2221, 21.4824) (-12.9741, -12.5756, 21.4824)
  arc A4 through (32.7346, -12.0756, 20.9824) (32.5881, -12.0756, 21.336) (32.2346, -12.0756, 21.4824)
  arc A5 through (32.2346, -12.0756, -3.3362) (32.5881, -12.0756, -3.1898) (32.7346, -12.0756, -2.8362)
  arc A6 through (31.8, -12.0756, -3.3362) (31.4464, -12.2221, -3.3362) (31.3, -12.5756, -3.3362)
  arc A7 through (-12.9741, -20.325, 3.7188) (-12.9741, -19.9714, 3.5724) (-12.9741, -19.825, 3.2188)
  circle A8 through (31.65, -16, 6.8238) (31.125, -16, 7.1269) (31.125, -16, 6.5207)
  circle A9 through (31.65, -16, 1.7438) (31.125, -16, 2.0469) (31.125, -16, 1.4407)
  circle A10 through (34.19, -16, -3.3362) (33.665, -16, -3.0331) (33.665, -16, -3.6393)
  circle A11 through (31.65, -16, -0.7962) (31.125, -16, -0.4931) (31.125, -16, -1.0993)
  circle A12 through (34.19, -16, 6.8238) (33.665, -16, 7.1269) (33.665, -16, 6.5207)
  circle A13 through (34.19, -16, -0.7962) (33.665, -16, -0.4931) (33.665, -16, -1.0993)
  circle A14 through (34.19, -16, -5.8762) (33.665, -16, -5.5731) (33.665, -16, -6.1793)
  circle A15 through (34.19, -16, 4.2838) (33.665, -16, 4.5869) (33.665, -16, 3.9807)
  circle A16 through (31.65, -16, -5.8762) (31.125, -16, -5.5731) (31.125, -16, -6.1793)
  circle A17 through (31.65, -16, -3.3362) (31.125, -16, -3.0331) (31.125, -16, -3.6393)
  circle A18 through (34.19, -16, 9.3638) (33.665, -16, 9.6669) (33.665, -16, 9.0607)
  circle A19 through (34.19, -16, 1.7438) (33.665, -16, 2.0469) (33.665, -16, 1.4407)
  circle A20 through (31.65, -16, 4.2838) (31.125, -16, 4.5869) (31.125, -16, 3.9807)
  circle A21 through (31.65, -16, 9.3638) (31.125, -16, 9.6669) (31.125, -16, 9.0607)
  dimension "d149" = 0.25
  dimension "d150" = 0.5
  dimension "d157" = 0.5
sketch "Sketch22" plane through (-14.3562, 0, 0) normal (-1, 0, 0) x (0, -1, 0)
  circle A0 centre (-19.0259, -19.825) radius 0.35
  line L0 (-19.0259, -19.825, 0) -> (-19.0259, -19.825, 1.0685)
  line L1 (-19.0259, -20.325, 1.5685) -> (-19.0259, -22.75, 1.5685)
  line L2 (-19.0259, -23.25, 2.0685) -> (-19.0259, -23.25, 21.8638)
  line L3 (33.84, -13.4533, 21.8638) -> (33.84, -13.4533, -2.8362)
  line L4 (33.84, -13.9533, -3.3362) -> (33.84, -16, -3.3362)
  line L5 (-19.0259, -22.75, 22.3638) -> (-19.0259, -13.9533, 22.3638)
  line L6 (-18.5259, -13.4533, 22.3638) -> (33.34, -13.4533, 22.3638)
  arc A1 through (-19.0259, -22.75, 22.3638) (-19.0259, -23.1036, 22.2173) (-19.0259, -23.25, 21.8638)
  arc A2 through (-18.5259, -13.4533, 22.3638) (-18.8795, -13.5997, 22.3638) (-19.0259, -13.9533, 22.3638)
  arc A3 through (-19.0259, -23.25, 2.0685) (-19.0259, -23.1036, 1.715) (-19.0259, -22.75, 1.5685)
  arc A4 through (-19.0259, -20.325, 1.5685) (-19.0259, -19.9714, 1.4221) (-19.0259, -19.825, 1.0685)
  arc A5 through (33.34, -13.4533, 22.3638) (33.6936, -13.4533, 22.2173) (33.84, -13.4533, 21.8638)
  arc A6 through (33.84, -13.9533, -3.3362) (33.84, -13.5997, -3.1898) (33.84, -13.4533, -2.8362)
  circle A7 through (31.65, -16, 6.8238) (31.125, -16, 7.1269) (31.125, -16, 6.5207)
  circle A8 through (31.65, -16, 1.7438) (31.125, -16, 2.0469) (31.125, -16, 1.4407)
  circle A9 through (34.19, -16, -3.3362) (33.665, -16, -3.0331) (33.665, -16, -3.6393)
  circle A10 through (31.65, -16, -0.7962) (31.125, -16, -0.4931) (31.125, -16, -1.0993)
  circle A11 through (34.19, -16, 6.8238) (33.665, -16, 7.1269) (33.665, -16, 6.5207)
  circle A12 through (34.19, -16, -0.7962) (33.665, -16, -0.4931) (33.665, -16, -1.0993)
  circle A13 through (34.19, -16, -5.8762) (33.665, -16, -5.5731) (33.665, -16, -6.1793)
  circle A14 through (34.19, -16, 4.2838) (33.665, -16, 4.5869) (33.665, -16, 3.9807)
  circle A15 through (31.65, -16, -5.8762) (31.125, -16, -5.5731) (31.125, -16, -6.1793)
  circle A16 through (31.65, -16, -3.3362) (31.125, -16, -3.0331) (31.125, -16, -3.6393)
  circle A17 through (34.19, -16, 9.3638) (33.665, -16, 9.6669) (33.665, -16, 9.0607)
  circle A18 through (34.19, -16, 1.7438) (33.665, -16, 2.0469) (33.665, -16, 1.4407)
  circle A19 through (31.65, -16, 4.2838) (31.125, -16, 4.5869) (31.125, -16, 3.9807)
  circle A20 through (31.65, -16, 9.3638) (31.125, -16, 9.6669) (31.125, -16, 9.0607)
  dimension "d158" = 0.25
  dimension "d159" = 0.5
  dimension "d166" = 9
equation "d2 = 15 mm + 4.06 mm - 0.31 mm"
equation "d10 = d9 / 2"
equation "d12 = d11 / 2"
